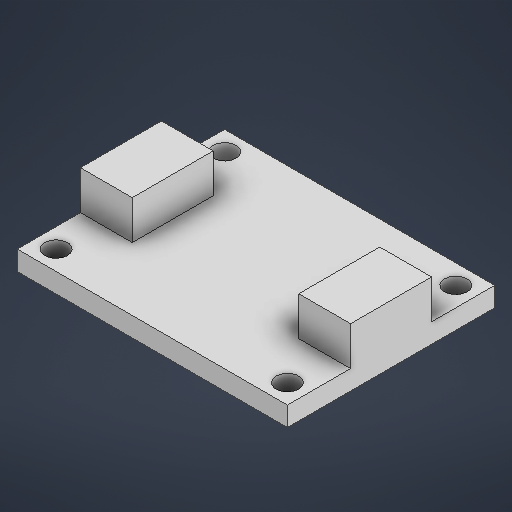
# Autodesk Inventor part: sensor conditioning board simplified model
Saved by Autodesk Inventor 2026 (Build 300175050, 175E)
## iProperties
Created: 2025-08-07
Part Number: sensor conditioning board simplified model
Material: Generic
Document SubType Name: Modeling
Designer: localuser
Density: 1 g/cm^3
Appearance: Default
Author: localuser
Autodesk Inventor part; units mm, degrees
ref_plane "YZ Plane" through (0, 0, 0) normal (1, 0, 0) x (0, 1, 0)
ref_plane "XZ Plane" through (0, 0, 0) normal (0, 1, 0) x (-1, 0, 0)
ref_plane "XY Plane" through (0, 0, 0) normal (0, 0, 1) x (1, 0, 0)
sketch "Sketch1" plane through (0, 0, 0) normal (0, 1, 0) x (-1, 0, 0)
  line L0 (0, 0) -> (0, -32)
  line L1 (0, -32) -> (41.7, -32)
  line L2 (41.7, -32) -> (41.7, 0)
  line L3 (41.7, 0) -> (0, 0)
  line L4 (41.7, 0) -> (38.7, 0)
  line L5 (38.7, 0) -> (38.7, -3)
  line L6 (0, 0) -> (0, -3)
  line L7 (0, -3) -> (3, -3)
  line L8 (0, -32) -> (0, -29)
  line L9 (0, -29) -> (3, -29)
  line L10 (41.7, -32) -> (38.7, -32)
  line L11 (38.7, -32) -> (38.7, -29)
  circle A0 centre (38.7, -3) radius 1.75
  circle A1 centre (38.7, -29) radius 1.75
  circle A2 centre (3, -3) radius 1.75
  circle A3 centre (3, -29) radius 1.75
  dimension "d0" = 32
  dimension "d1" = 41.7
  dimension "d2" = 32
  dimension "d3" = 3
  dimension "d4" = 3
  dimension "d5" = 3
  dimension "d6" = 3
  dimension "d7" = 3
  dimension "d8" = 3
  dimension "d9" = 3
  dimension "d10" = 3
  dimension "d11" = 3.5
  dimension "d12" = 3.5
  dimension "d13" = 3.5
  constraints: 24 end point, 5 perpendicular, 4 centre point, 4 coincident, 4 point on line, 1 horizontal, 1 vertical
  measures "d0" distance of L0.start L0.end
  measures "d1" distance of L0.end L1.end
  measures "d2" distance of L1.end L2.end
  measures "d3" distance of L2.end L4.end
  measures "d4" distance of L4.end L5.end
  measures "d5" distance of L0.start L6.end
  measures "d6" distance of L6.end L7.end
  measures "d7" distance of L0.end L8.end
  measures "d8" distance of L8.end L9.end
  measures "d9" distance of L1.end L10.end
  measures "d10" distance of L10.end L11.end
  measures "d11" diameter of A0
  measures "d12" diameter of A1
  measures "d13" diameter of A3
extrude "Extrusion1" add sketch "Sketch1" along normal blind 3
sketch "Sketch2" plane through (0, 3, 0) normal (0, 1, 0) x (1, 0, 0)
  line L0 (0, 0) -> (0, 32) projected
  line L1 (0, 0) -> (0, 32)
  line L2 (0, 32) -> (0, 16)
  line L3 (0, 16) -> (0, 22.25)
  line L4 (0, 22.25) -> (-41.7, 22.25)
  line L5 (-41.7, 22.25) -> (-41.7, 9.75)
  line L6 (-41.7, 9.75) -> (0, 9.75)
  line L7 (0, 9.75) -> (0, 16)
  line L8 (0, 9.75) -> (-8, 9.75)
  line L9 (-8, 9.75) -> (-8, 22.25)
  line L10 (-8, 22.25) -> (0, 22.25)
  line L11 (-41.7, 22.25) -> (-33.7, 22.25)
  line L12 (-33.7, 22.25) -> (-33.7, 9.75)
  line L13 (-41.7, 9.75) -> (-33.7, 9.75)
  dimension "d16" = 6.25
  dimension "d17" = 41.7
  dimension "d18" = 12.5
  dimension "d19" = 8
  dimension "d20" = 8
  constraints: 26 end point, 7 perpendicular, 6 point on line, 1 collinear, 1 midpoint, 1 vertical
  measures "d16" distance of L2.end L3.end
  measures "d17" distance of L3.end L4.end
  measures "d18" distance of L4.end L5.end
  measures "d19" distance of L6.end L8.end
  measures "d20" distance of L4.end L11.end
extrude "Extrusion2" add sketch "Sketch2" along normal blind 6 contours L6 L9 L4 L0 | L6 L5 L4 L12
body "Solid1"
